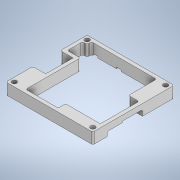
# Autodesk Inventor part: SPI-Buffer-Interposer
Saved by Autodesk Inventor 2020.3 (Build 243373000, 373)
## iProperties
Created: 2020-05-27
Part Number: SPI-Buffer-Interposer
Material: Generic
Document SubType Name: Modeling
Designer: User
Density: 1 g/cm^3
Appearance: Default
Author: User
Autodesk Inventor part; units mm, degrees
ref_plane "YZ Plane" through (0, 0, 0) normal (1, 0, 0) x (0, 1, 0)
ref_plane "XZ Plane" through (0, 0, 0) normal (0, 1, 0) x (-1, 0, 0)
ref_plane "XY Plane" through (0, 0, 0) normal (0, 0, 1) x (1, 0, 0)
sketch "Sketch1" plane through (0, 0, 0) normal (0, 1, 0) x (-1, 0, 0)
  line L0 (-23.6538, 22.098) -> (23.6538, 22.098)
  line L1 (23.6538, 22.098) -> (23.6538, -22.098)
  line L2 (23.6538, -22.098) -> (-23.6538, -22.098)
  line L3 (-23.6538, -22.098) -> (-23.6538, 22.098)
  line L4 (-23.6538, 22.098) -> (23.6538, -22.098) construction
  line L5 (23.6538, 22.098) -> (-23.6538, -22.098) construction
  line L6 (23.6537, -7.493) -> (-23.6538, -7.493) construction
  line L7 (23.6537, 7.493) -> (-23.6538, 7.493) construction
  line L8 (16.6687, 22.098) -> (16.6688, -22.098) construction
  line L9 (23.6537, 7.493) -> (16.6687, 7.493)
  line L10 (16.6687, -7.493) -> (23.6537, -7.493)
  line L11 (16.6687, -7.493) -> (16.6687, 7.493)
  line L12 (23.6538, -22.098) -> (19.2723, -22.098) construction
  line L13 (19.2723, -22.098) -> (19.2723, -17.7165) construction
  line L14 (19.2723, -17.7165) -> (23.6538, -17.7165) construction
  line L15 (23.6538, -17.7165) -> (23.6538, -22.098) construction
  line L16 (23.6538, 22.098) -> (19.2723, 22.098) construction
  line L17 (19.2723, 22.098) -> (19.2723, 17.7165) construction
  line L18 (19.2723, 17.7165) -> (23.6538, 17.7165) construction
  line L19 (23.6538, 17.7165) -> (23.6538, 22.098) construction
  line L20 (-23.6538, 22.098) -> (-19.2723, 22.098) construction
  line L21 (-19.2723, 22.098) -> (-19.2723, 17.7165) construction
  line L22 (-19.2723, 17.7165) -> (-23.6538, 17.7165) construction
  line L23 (-23.6538, 17.7165) -> (-23.6538, 22.098) construction
  line L24 (-23.6538, -22.098) -> (-19.2723, -22.098) construction
  line L25 (-19.2723, -22.098) -> (-19.2723, -17.7165) construction
  line L26 (-19.2723, -17.7165) -> (-23.6538, -17.7165) construction
  line L27 (-23.6538, -17.7165) -> (-23.6538, -22.098) construction
  circle A0 centre (21.3678, 19.812) radius 1.27
  circle A1 centre (-21.3678, 19.812) radius 1.27
  circle A2 centre (-21.3678, -19.812) radius 1.27
  circle A3 centre (21.3678, -19.812) radius 1.27
  line L28 (21.7487, -20.193) -> (21.7487, 20.193) construction
  line L29 (21.7487, 20.193) -> (-21.7487, 20.193) construction
  line L30 (-21.7487, 20.193) -> (-21.7487, -20.193) construction
  line L31 (-21.7487, -20.193) -> (21.7487, -20.193) construction
  line L32 (23.6538, 9.398) -> (14.7637, 9.398) construction
  line L33 (14.7637, 9.398) -> (14.7637, -9.398) construction
  line L34 (14.7637, -9.398) -> (23.6538, -9.398) construction
  line L35 (21.7487, 9.398) -> (21.7487, 17.7165)
  line L36 (21.7487, 17.7165) -> (19.2723, 17.7165)
  line L37 (19.2723, 17.7165) -> (19.2723, 20.193)
  line L38 (19.2723, 20.193) -> (-19.2722, 20.193)
  line L39 (-19.2722, 20.193) -> (-19.2723, 17.7165)
  line L40 (-19.2723, 17.7165) -> (-21.7487, 17.7165)
  line L41 (-21.7487, 17.7165) -> (-21.7487, -17.7165)
  line L42 (-21.7487, -17.7165) -> (-19.2723, -17.7165)
  line L43 (-19.2723, -17.7165) -> (-19.2723, -20.193)
  line L44 (-19.2723, -20.193) -> (19.2722, -20.193)
  line L45 (19.2722, -20.193) -> (19.2723, -17.7165)
  line L46 (19.2723, -17.7165) -> (21.7487, -17.7165)
  line L47 (21.7487, -17.7165) -> (21.7487, -9.398)
  line L48 (21.7487, -9.398) -> (14.7637, -9.398)
  line L49 (14.7637, -9.398) -> (14.7637, 9.398)
  line L50 (14.7637, 9.398) -> (21.7487, 9.398)
  line L51 (14.7637, 9.398) -> (14.7637, 20.193)
  line L52 (-21.7487, 16.1417) -> (-2.8258, 16.1417)
  line L53 (-2.8258, 16.1417) -> (-2.8258, 20.193)
  line L54 (-21.7487, -5.0165) -> (-16.0338, -5.0165)
  line L55 (-16.0338, -5.0165) -> (-16.0337, -20.193)
  point P0 (0, 0)
  dimension "d0" = 47.3075
  dimension "d1" = 44.196
  dimension "d2" = 14.605
  dimension "d3" = 14.605
  dimension "d4" = 6.985
  dimension "d5" = 4.3815
  dimension "d6" = 4.3815
  dimension "d7" = 4.3815
  dimension "d8" = 4.3815
  dimension "d9" = 4.3815
  dimension "d10" = 4.3815
  dimension "d11" = 4.3815
  dimension "d12" = 4.3815
  dimension "d13" = 2.54
  dimension "d14" = 2.54
  dimension "d15" = 2.54
  dimension "d16" = 2.54
  dimension "d17" = 2.286
  dimension "d18" = 2.286
  dimension "d19" = 2.286
  dimension "d20" = 2.286
  dimension "d21" = 2.286
  dimension "d22" = 2.286
  dimension "d23" = 2.286
  dimension "d24" = 2.286
  dimension "d25" = 1.905
  dimension "d26" = 1.905
  dimension "d27" = 1.905
  dimension "d28" = 1.905
  dimension "d46" = 5.9563
  dimension "d47" = 20.828
  dimension "d48" = 17.0815
  dimension "d49" = 7.62
  constraints: 112 end point, 37 point on line, 17 perpendicular, 12 parallel, 8 horizontal, 6 collinear, 4 centre point, 2 midpoint, 3 other
  measures "d0" distance of L1.end L2.end
  measures "d1" distance of L0.end L1.end
  measures "d2" distance between parallel lines of L2 L6
  measures "d3" distance between parallel lines of L0 L7
  measures "d4" distance between parallel lines of L1 L8
  measures "d5" distance of L13.end L14.end
  measures "d6" distance of L12.end L13.end
  measures "d7" distance of L18.end L17.end
  measures "d8" distance of L17.end L16.end
  measures "d9" distance of L21.end L22.end
  measures "d10" distance of L20.end L21.end
  measures "d11" distance of L26.end L25.end
  measures "d12" distance of L25.end L24.end
  measures "d13" diameter of A0
  measures "d14" diameter of A1
  measures "d15" diameter of A2
  measures "d16" diameter of A3
  measures "d17" distance from line of L0 A0.centre
  measures "d18" distance from line of L12 A3.centre
  measures "d19" distance from line of L2 A2.centre
  measures "d20" distance from line of L0 A1.centre
  measures "d21" distance from line of L3 A1.centre
  measures "d22" distance from line of L1 A0.centre
  measures "d23" distance from line of L15 A3.centre
  measures "d24" distance from line of L3 A2.centre
  measures "d25" distance between parallel lines of L1 L28
  measures "d26" distance between parallel lines of L34 L6
  measures "d27" distance between parallel lines of L33 L11
  measures "d28" distance between parallel lines of L32 L9
  measures "d46" distance between parallel lines of L0 L52
  measures "d47" distance between parallel lines of L3 L53
  measures "d48" distance between parallel lines of L2 L54
  measures "d49" distance between parallel lines of L3 L55
extrude "Extrusion1" add sketch "Sketch1" along normal blind 6.02 contours L0 L1 L9 L11 L10 L2 L3 | L50 L51 L38 L37 L36 L35 | L53 L52 L41 L40 L39 L38 | L54 L55 L44 L43 L42 L41
sketch "Sketch2" plane through (23.6538, 0, 22.098) normal (1, 0, 0) x (0, 0, -1)
  line L0 (16.0782, 0) -> (27.0002, 0)
  line L1 (27.0002, 0) -> (27.0002, 3.175)
  line L2 (27.0002, 3.175) -> (16.0782, 3.175)
  line L3 (16.0782, 3.175) -> (16.0782, 0)
  line L4 (44.196, 0) -> (44.196, 6.02) projected
  line L5 (0, 0) -> (44.196, 0) projected
  line L6 (16.0782, 2.4257) -> (7.7597, 2.4257)
  line L7 (7.7597, 2.4257) -> (7.7597, 0)
  line L8 (7.7597, 0) -> (16.0782, 0)
  line L9 (16.0782, 0) -> (16.0782, 2.4257)
  point P0 (22.098, 0)
  point P1 (7.7597, 0)
  dimension "d31" = 10.922
  dimension "d32" = 3.175
  dimension "d33" = 17.1958
  dimension "d34" = 8.3185
  dimension "d35" = 2.4257
  constraints: 16 end point, 4 parallel, 2 collinear, 2 horizontal, 2 perpendicular, 1 point on line
  measures "d31" distance of L2.end L1.end
  measures "d32" distance of L1.end L0.end
  measures "d33" distance between parallel lines of L1 L4
  measures "d34" distance of L8.end L7.end
  measures "d35" distance of L7.end L6.end
extrude "Extrusion2" cut sketch "Sketch2" against normal blind 25.4
sketch "Sketch3" plane through (23.6538, 0, -22.098) normal (0, 0, -1) x (-1, 0, 0)
  line L0 (42.926, 0) -> (45.4025, 0) projected
  line L1 (42.2021, 0) -> (39.5351, 0)
  line L2 (39.5351, 0) -> (39.5351, 0.8382)
  line L3 (39.5351, 0.8382) -> (42.2021, 0.8382)
  line L4 (42.2021, 0.8382) -> (42.2021, 0)
  line L5 (20.828, 0) -> (38.4175, 0) projected
  line L6 (26.8605, 0) -> (29.5275, 0)
  line L7 (29.5275, 0) -> (29.5275, 0.8382)
  line L8 (29.5275, 0.8382) -> (26.8605, 0.8382)
  line L9 (26.8605, 0.8382) -> (26.8605, 0)
  line L10 (47.3075, 0) -> (47.3075, 6.02) projected
  line L11 (0, 0) -> (0, 6.02) projected
  point P0 (23.6538, 0)
  point P1 (4.3815, 0)
  dimension "d38" = 2.667
  dimension "d39" = 0.8382
  dimension "d40" = 2.667
  dimension "d41" = 0.8382
  dimension "d42" = 5.1054
  dimension "d43" = 26.8605
  constraints: 16 end point, 4 parallel, 2 horizontal, 2 perpendicular, 2 point on line
  measures "d38" distance of L2.end L3.end
  measures "d39" distance of L1.end L2.end
  measures "d40" distance of L8.end L7.end
  measures "d41" distance of L7.end L6.end
  measures "d42" distance between parallel lines of L10 L4
  measures "d43" distance between parallel lines of L11 L9
extrude "Extrusion3" cut sketch "Sketch3" against normal up to next
move faces "Move1" translate (0, 0, 0.1143) faces at (17.9387, 2.0067, -5.0165)
fillet "Fillet1" radius 0.9525 19 edges at (23.6538, 3.01, -22.098) (-23.6538, 3.01, -22.098) (-23.6537, 3.01, -7.493) (-16.6687, 3.01, 7.493) (-23.6537, 3.01, 7.493) (-23.6538, 3.01, 22.098) (23.6538, 3.01, 22.098) (-14.7637, 3.01, -9.398) (-21.7487, 3.01, -9.398) (-19.2723, 3.01, -17.7165) (2.8258, 3.01, 16.1417) (2.8258, 3.01, 20.193) (21.7487, 3.01, 16.1417) (-14.7637, 3.01, 20.193) (16.0338, 3.01, -4.9022) (16.0337, 3.01, -20.193) (-19.2722, 3.01, -20.193) (-21.7487, 3.01, -17.7165) (21.7487, 4.5975, -4.9022)
fillet "Fillet3" radius 0.35 2 edges at (22.7012, 2.4257, 6.0198) (22.7012, 3.175, 6.0198)
fillet "Fillet4" radius 0.9525 3 edges at (22.7012, 2.4257, 14.3383) (21.2725, 3.175, -4.9022) (22.7012, 3.175, -4.9022)
fillet "Fillet5" radius 0.35 4 edges at (-3.2067, 0.8382, -21.1455) (-5.8738, 0.8382, -21.1455) (-15.8814, 0.8382, -21.1455) (-18.5484, 0.8382, -21.1316)
equation "\"d26\" = d25"
equation "\"d27\" = d25"
equation "\"d28\" = d25"
body "Solid1"
